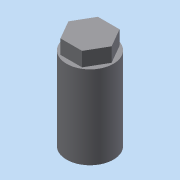
# Autodesk Inventor part: wheel connector
Saved by Autodesk Inventor 2015 (Build 190159000, 159)
## iProperties
Created: 2015-06-25
Part Number: wheel connector
Material: Generic
Document SubType Name: Modeling
Designer: Rahul
Density: 1 g/cm^3
Appearance: Default
Author: Rahul
Autodesk Inventor part; units mm, degrees
ref_plane "YZ Plane" through (0, 0, 0) normal (1, 0, 0) x (0, 1, 0)
ref_plane "XZ Plane" through (0, 0, 0) normal (0, 1, 0) x (-1, 0, 0)
ref_plane "XY Plane" through (0, 0, 0) normal (0, 0, 1) x (1, 0, 0)
sketch "Sketch1" plane through (0, 0, 0) normal (0, 1, 0) x (-1, 0, 0)
  line L0 (-3.4641, -6) -> (-6.9282, 0)
  line L1 (-6.9282, 0) -> (-3.4641, 6)
  line L2 (-3.4641, 6) -> (3.4641, 6)
  line L3 (3.4641, 6) -> (6.9282, 0)
  line L4 (6.9282, 0) -> (3.4641, -6)
  line L5 (3.4641, -6) -> (-3.4641, -6)
  line L6 (10.5, 0) -> (-10.5, 0) projected
  line L7 (0, -10.5) -> (0, 10.5) projected
  circle A0 centre (0, 0) radius 2
  arc A1 (0.4459, -1.9497) -> (0.4459, -1.9497) centre (0, 0) ccw
  line L8 (1.64, 1.1447) -> (-1.64, 1.1447)
  circle A2 centre (0, 0) radius 2.025
  circle A3 centre (0, 0) radius 7.5
  dimension "d2" = 4
  dimension "d6" = 4.05
  dimension "d33" = 15
  dimension "d36" = 3.28
  dimension "d37" = 12
  constraints: 14 end point, 6 point on circle, 5 coincident, 4 centre point, 1 horizontal, 1 midpoint, 14 other
  measures "d2" diameter of A0
  measures "d6" diameter of A2
  measures "d33" diameter of A3
  measures "d36" distance of L8.start L8.end
  measures "d37" distance between parallel lines of L5 L2
extrude "Extrusion1" add sketch "Sketch1" along normal blind 4.57 contours L0 L6 A2 L7 L5 | L1 L2 L7 A2 L6 | L7 A2 L6 L4 L5 | L6 A0 L7 A2 | L7 A0 L6 A2 | L2 L3 L6 A2 L7 picked at (-1.8669, -0.7323) picked at (1.9162, -0.5914)
extrude "Extrusion6" add sketch "Sketch1" along normal blind 4.572 contours A2 L7 A0 L6 | L6 A0 L7 A2 | L7 A0 L6 A2 | A0 L8 L7 L6 | L6 L7 A0 | A2 L6 A0 L7 | L7 L6 A0 | L7 L8 A0 L6 | A0 L7 L8 | A0 L8 L7
extrude "Extrusion11" add sketch "Sketch1" against normal blind 17.8 contours A2 L7 A0 L6 | L6 A0 L7 A2 | L7 A0 L6 A2 | A0 L8 L7 L6 | L6 L7 A0 | A2 L6 A0 L7 | L7 L6 A0 | L7 L8 A0 L6 | A0 L7 L8 | A0 L8 L7
extrude "Extrusion12" add sketch "Sketch1" against normal blind 26.6 contours A2 L7 A0 L6 | A2 L6 A0 L7 | A0 L7 L8 | A0 L8 L7 picked at (-1.5145, 1.3032) picked at (1.5145, 1.3032)
extrude "Extrusion13" add sketch "Sketch1" against normal blind 26.6 contours L5 L7 A3 L6 L0 | L0 L6 A2 L7 L5 | L6 A3 L7 L2 L1 | L1 L2 L7 A2 L6 | L7 A2 L6 L4 L5 | L5 L4 L6 A3 L7 | L7 A3 L6 L3 L2 | L2 L3 L6 A2 L7
body "Solid1"
